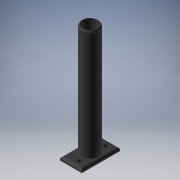
# Autodesk Inventor part: Flag Holder
Saved by Autodesk Inventor 2019 (Build 230136000, 136)
## iProperties
Created: 2019-01-10
Part Number: Flag Holder
Material: Generic
Document SubType Name: Modeling
Designer: Ashley
Density: 1 g/cm^3
Appearance: Default
Author: Ashley
Autodesk Inventor part; units mm, degrees
ref_plane "YZ Plane" through (0, 0, 0) normal (1, 0, 0) x (0, 1, 0)
ref_plane "XZ Plane" through (0, 0, 0) normal (0, 1, 0) x (-1, 0, 0)
ref_plane "XY Plane" through (0, 0, 0) normal (0, 0, 1) x (1, 0, 0)
sketch "Sketch1" plane through (0, 0, 0) normal (0, 1, 0) x (-1, 0, 0)
  circle A0 centre (5.2854, 6.2781) radius 7.75
  point P0 (0, 0)
  dimension "d0" = 15.5
  constraints: 1 centre point
  measures "d0" diameter of A0
extrude "Extrusion1" add sketch "Sketch1" along normal blind 101.6
sketch "Sketch2" plane through (-5.2854, 101.6, 6.2781) normal (0, 1, 0) x (1, 0, 0)
  circle A0 centre (0, 0) radius 7.75 construction
  circle A1 centre (0, 0) radius 7
  point P0 (5.2854, 6.2781)
  dimension "d3" = 14
  dimension "d4" = 0
  constraints: 1 centre point
  measures "d3" diameter of A1
  measures "d4" distance of A0.centre A1.centre
extrude "Extrusion2" cut sketch "Sketch2" against normal blind 101.6
sketch "Sketch3" plane through (-5.2854, 0, 6.2781) normal (0, -1, 0) x (1, 0, 0)
  circle A0 centre (0, 0) radius 7 construction
  line L0 (10, 17.5) -> (-10, 17.5)
  line L1 (-10, 17.5) -> (-10, -17.5)
  line L2 (-10, -17.5) -> (10, -17.5)
  line L3 (10, -17.5) -> (10, 17.5)
  circle A1 centre (2.5, 12) radius 2
  circle A2 centre (2.5, -12) radius 2
  point P0 (5.2854, -6.2781)
  dimension "d7" = 35
  dimension "d8" = 20
  dimension "d11" = 17.5
  dimension "d12" = 10
  dimension "d14" = 4
  dimension "d15" = 4
  dimension "d16" = 24
  dimension "d17" = 5.5
  dimension "d18" = 7.5
  dimension "d19" = 7.5
  constraints: 8 end point, 2 centre point, 2 parallel, 1 horizontal, 1 perpendicular
  measures "d7" distance of L2.end L0.start
  measures "d8" distance of L1.end L2.end
  measures "d11" distance from line of A0.centre L2
  measures "d12" distance from line of A0.centre L3
  measures "d14" diameter of A1
  measures "d15" diameter of A2
  measures "d16" distance of A2.centre A1.centre
  measures "d17" distance from line of L0 A1.centre
  measures "d18" distance from line of L3 A2.centre
  measures "d19" distance from line of L3 A1.centre
extrude "Extrusion3" add sketch "Sketch3" along normal blind 3
fillet "Fillet1" radius 2 4 edges at (-5.2854, 0, 23.7781) (-15.2854, 0, 6.2781) (-5.2854, 0, -11.2219) (4.7146, 0, 6.2781)
fillet "Fillet2" radius 2 1 edges at (2.4646, 101.6, 6.2781)
body "Solid1"
